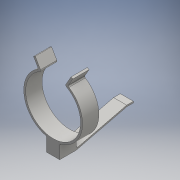
# Autodesk Inventor part: omikuji
Saved by Autodesk Inventor 2016 (Build 200138000, 138)
## iProperties
Created: 2016-06-10
Part Number: omikuji
Material: Générique
Document SubType Name: Modeling
Designer: Ropert
Density: 1 g/cm^3
Appearance: Par défaut
Author: Ropert
Autodesk Inventor part; units mm, degrees
ref_plane "YZ Plane" through (0, 0, 0) normal (1, 0, 0) x (0, 1, 0)
ref_plane "XZ Plane" through (0, 0, 0) normal (0, 1, 0) x (-1, 0, 0)
ref_plane "XY Plane" through (0, 0, 0) normal (0, 0, 1) x (1, 0, 0)
sketch "Esquisse1" plane through (0, 0, 0) normal (0, 1, 0) x (-1, 0, 0)
  line L0 (22.5, 38.9711) -> (30, 51.9615)
  line L1 (0, 0) -> (55, 0) construction
  line L2 (-22.5, 38.9711) -> (-30, 51.9615)
  line L3 (0, 0) -> (55, 0) construction
  line L4 (0, -65) -> (10, -65)
  line L5 (10, -65) -> (10, -43.8748)
  line L6 (0, -65) -> (-10, -65)
  line L7 (-10, -65) -> (-10, -43.8748)
  line L8 (27.4019, 53.4615) -> (18.3483, 37.7802)
  arc A0 (-18.3483, 37.7802) -> (18.3483, 37.7802) centre (0, 0) ccw
  line L9 (-18.3483, 37.7802) -> (-27.4019, 53.4615)
  line L10 (27.4019, 53.4615) -> (30, 51.9615)
  line L11 (-30, 51.9615) -> (-27.4019, 53.4615)
  arc A1 (-22.5, 38.9711) -> (-10, -43.8748) centre (0, 0) ccw
  arc A2 (10, -43.8748) -> (22.5, 38.9711) centre (0, 0) ccw
  dimension "d1" = 60
  dimension "d2" = 60
  dimension "d3" = 60
  dimension "d4" = 120
  constraints: 24 end point, 6 point on circle, 4 horizontal, 3 centre point, 1 coincident, 1 perpendicular
  measures "d1" distance of L1.start L0.end
  measures "d2" angle of L1 L0
  measures "d3" distance of L1.start L2.end
  measures "d4" angle of L3 L2
extrude "Extrusion1" add sketch "Esquisse1" along normal blind 25
sketch "Esquisse2" plane through (10, 0, -43.8748) normal (1, 0, 0) x (0, 0, -1)
  line L0 (0, 25) -> (21.1252, 25) projected
  line L1 (21.1252, 25) -> (2.2112, 102.732)
  line L2 (2.2112, 102.732) -> (2.2112, 112.732)
  line L3 (0, 112.732) -> (0, 102.4668)
  line L4 (0, 102.4668) -> (18.8494, 25)
  line L5 (0, 112.732) -> (2.2112, 112.732)
  point P0 (-43.8748, 0)
  dimension "d11" = 80
  dimension "d12" = 10
  constraints: 10 end point, 1 horizontal, 1 perpendicular, 1 point on line
  measures "d11" distance of L0.end L1.end
  measures "d12" distance of L1.end L2.end
extrude "Extrusion2" add sketch "Esquisse2" against normal blind 20
fillet "Congé1" radius 2 1 edges at (0, 25, -62.7243)
fillet "Congé2" radius 2 2 edges at (10, 12.5, -43.8748) (-10, 12.5, -43.8748)
fillet "Congé3" radius 2 4 edges at (18.3483, 12.5, 37.7802) (-18.3483, 12.5, 37.7802) (22.5, 12.5, 38.9711) (-22.5, 12.5, 38.9711)
